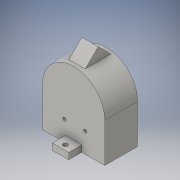
# Autodesk Inventor part: Tail5
Saved by Autodesk Inventor 2016 (Build 200138000, 138)
## iProperties
Created: 2017-03-09
Part Number: Tail5
Material: Generic
Document SubType Name: Modeling
Designer: Owner
Density: 1 g/cm^3
Appearance: Default
Author: Owner
Autodesk Inventor part; units mm, degrees
ref_plane "YZ Plane" through (0, 0, 0) normal (1, 0, 0) x (0, 1, 0)
ref_plane "XZ Plane" through (0, 0, 0) normal (0, 1, 0) x (-1, 0, 0)
sketch "Sketch1" plane through (0, 0, 0) normal (0, 0, 1) x (1, 0, 0)
  line L0 (-21.6147, -38.1) -> (42.5469, -38.1) projected
  line L1 (6.35, -38.0962) -> (6.35, -43.1) projected
  line L2 (6.35, -43.1) -> (22.86, -43.1) projected
  line L3 (22.86, -43.1) -> (22.86, 0) projected
  arc A0 (22.86, 0) -> (-22.86, 0) centre (0, 0) ccw projected
  line L4 (-22.86, 0) -> (-22.86, -43.1) projected
  line L5 (-22.86, -43.1) -> (-6.35, -43.1) projected
  line L6 (-6.35, -43.1) -> (-6.35, -38.0962) projected
  line L7 (-6.35, -38.0962) -> (6.35, -38.0962) projected
  line L8 (17.78, -43.1) -> (-24.13, -43.1)
  line L9 (-24.13, -43.1) -> (24.13, -43.1)
  line L10 (0, 0) -> (0, -12.7)
  circle A1 centre (0, -12.7) radius 24.13
  line L11 (-24.13, -12.7) -> (24.13, -12.7)
  line L12 (24.13, -12.7) -> (24.13, -43.1)
  line L13 (24.13, -43.1) -> (-24.13, -43.1)
  line L14 (-24.13, -43.1) -> (-24.13, -12.7)
  dimension "d20" = 48.26
  dimension "d19" = 12.7
  constraints: 14 end point, 2 coincident, 2 horizontal, 2 parallel, 1 horizontal alignment, 1 perpendicular, 1 point on line, 1 vertical, 2 other
  measures "d19" distance of L10.start L10.end
extrude "Extrusion1" add sketch "Sketch1" along normal blind 25.4 contours L6 L7 L1 L0 | L0 L1 L8 L6 | L6 L5 L4 A1 L3 L0 L1 L7 | L0 L3 L2 L1 | L3 A1 L12 L0 | L0 L12 L9 L3 | L8 L14 A1 L4 | A1 L4 L11 L3 | L3 L11 A1 | A1 L11 L4 | L11 L3 A1 | L11 L4 A1 L3 | L11 A1 L4
sketch "Sketch2" plane through (0, 0, 0) normal (0, 0, -1) x (-1, 0, 0)
  line L0 (6.35, -43.1) -> (-6.35, -43.1) projected
  line L1 (-6.35, -43.1) -> (-6.35, -38.0962) projected
  line L2 (-6.35, -38.0962) -> (6.35, -38.0962) projected
  line L3 (6.35, -38.0962) -> (6.35, -43.1) projected
  line L4 (6.35, -38.0962) -> (-6.35, -38.0962)
  line L5 (-6.35, -38.0962) -> (-6.35, -33.0924)
  line L6 (-6.35, -33.0924) -> (6.35, -33.0924)
  line L7 (6.35, -33.0924) -> (6.35, -38.0962)
  point P0 (0, 0)
  dimension "d3" = 5.0038
  constraints: 8 end point, 2 parallel, 1 horizontal, 1 perpendicular
  measures "d3" distance of L6.end L2.end
extrude "Extrusion2" add sketch "Sketch2" along normal blind 10.16 contours L2 L5 L6 L7
sketch "Sketch3" plane through (-6.35, -33.0924, 0) normal (0, 1, 0) x (1, 0, 0)
  line L0 (12.7, 10.16) -> (0, 10.16) projected
  line L1 (6.35, 10.16) -> (6.35, 6.35)
  circle A0 centre (6.35, 6.35) radius 2.25
  point P0 (6.35, 0)
  dimension "d6" = 3.81
  dimension "d7" = 4.5
  constraints: 2 end point, 1 centre point, 1 coincident, 1 midpoint, 1 vertical
  measures "d6" distance of L1.start L1.end
  measures "d7" diameter of A0
extrude "Extrusion3" cut sketch "Sketch3" against normal blind 10.16
sketch "Sketch4" plane through (0, 0, 25.4) normal (0, 0, 1) x (1, 0, 0)
  line L0 (0, -43.1) -> (6.35, -43.1)
  line L1 (6.35, -43.1) -> (-6.35, -43.1)
  line L2 (-6.35, -43.1) -> (6.35, -43.1)
  line L3 (6.35, -43.1) -> (6.35, -38.0962)
  line L4 (6.35, -38.0962) -> (-6.35, -38.0962)
  line L5 (-6.35, -38.0962) -> (-6.35, -43.1)
  point P0 (0, 0)
  dimension "d10" = 6.35
  dimension "d11" = 12.7
  dimension "d12" = 5.0038
  constraints: 12 end point, 2 parallel, 1 horizontal, 1 perpendicular
  measures "d10" distance of L0.start L0.end
  measures "d11" distance of L0.end L1.end
  measures "d12" distance of L2.end L3.end
extrude "Extrusion4" add sketch "Sketch4" along normal blind 10.16
sketch "Sketch5" plane through (-6.35, -38.0962, 25.4) normal (0, 1, 0) x (1, 0, 0)
  line L0 (0, -10.16) -> (12.7, -10.16) projected
  line L1 (6.35, -10.16) -> (6.35, -6.35)
  circle A0 centre (6.35, -6.35) radius 1.75
  point P0 (6.35, 25.4)
  dimension "d15" = 3.81
  dimension "d16" = 3.5
  constraints: 2 end point, 1 centre point, 1 coincident, 1 midpoint, 1 vertical
  measures "d15" distance of L1.start L1.end
  measures "d16" diameter of A0
extrude "Extrusion5" cut sketch "Sketch5" against normal blind 10.16
ref_plane "Work Plane1" through (0, -43.1, 0) normal (-1, 0, 0) x (0, 0, 1)
sketch "Sketch6" plane through (0, -43.1, 0) normal (-1, 0, 0) x (0, 0, 1)
  line L0 (0, 54.53) -> (0, 30.4) projected
  line L1 (0, 54.53) -> (2.7051, 54.53)
  line L2 (0, 54.53) -> (25.4, 54.53) projected
  line L3 (2.7051, 54.53) -> (22.6949, 54.53)
  line L4 (22.6949, 54.53) -> (12.6873, 54.53)
  line L5 (12.6873, 54.53) -> (12.6873, 64.5376)
  line L6 (12.6873, 64.5376) -> (22.6949, 54.53)
  line L7 (12.6873, 64.5376) -> (2.7051, 54.53)
  point P0 (0, 43.1)
  dimension "d22" = 2.7051
  dimension "d23" = 19.9898
  dimension "d24" = 10.0076
  dimension "d25" = 10.0076
  constraints: 12 end point, 3 point on line, 1 perpendicular
  measures "d22" distance of L0.start L1.end
  measures "d23" distance of L1.end L3.end
  measures "d24" distance of L3.end L4.end
  measures "d25" distance of L4.end L5.end
extrude "Extrusion6" add sketch "Sketch6" along normal mid plane 12.7
sketch "Sketch7" plane through (0, 0, 0) normal (0, 0, -1) x (-1, 0, 0)
  ellipse E0 centre (-10.0535, -27.5683) end of major axis (-10.0535, -26.3237) minor radius 1.2444 projected
  ellipse E1 centre (8.0741, -27.5683) end of major axis (8.0741, -26.3237) minor radius 1.2444 projected
  line L0 (-10.0535, -27.5683) -> (-9.0535, -27.5683)
  circle A0 centre (-9.0535, -27.5683) radius 1.2446
  line L1 (8.0741, -27.5683) -> (7.0741, -27.5683)
  circle A1 centre (7.0741, -27.5683) radius 1.2446
  point P0 (0, 0)
  dimension "d28" = 1
  dimension "d29" = 2.4892
  dimension "d30" = 1
  dimension "d31" = 2.4892
  constraints: 4 end point, 2 centre point, 2 coincident, 2 horizontal, 2 other
  measures "d28" distance of L0.start L0.end
  measures "d29" diameter of A0
  measures "d30" distance of L1.start L1.end
  measures "d31" diameter of A1
extrude "Extrusion7" cut sketch "Sketch7" against normal blind 25.4 contours A0 E0 | E0 A0 | A1 E1 | E1 A1 picked at (-9.7984, -27.3936) picked at (-8.155, -27.4665) picked at (7.819, -27.743) picked at (6.1756, -27.6701)
body "Solid1"
